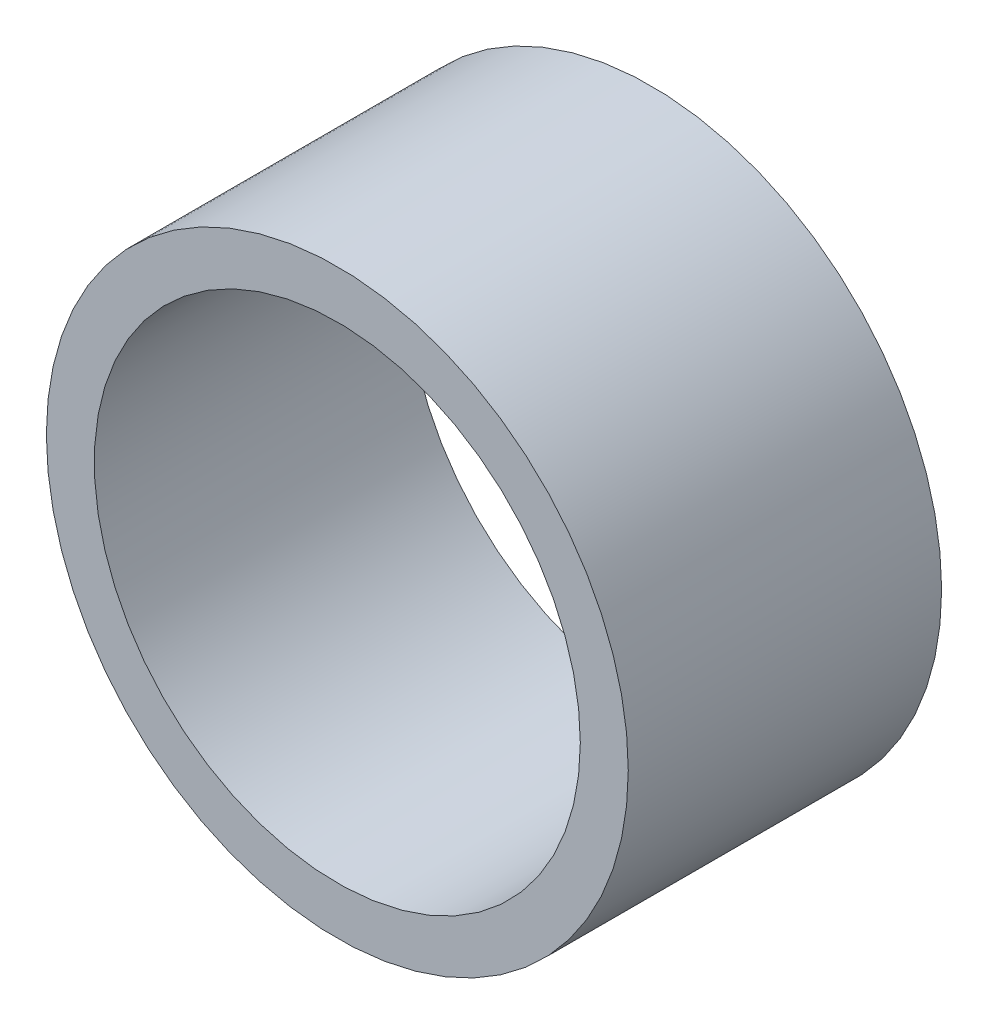
# Autodesk Inventor part: spacer for top of drivetrain
Saved by Autodesk Inventor 2020 (Build 240168000, 168)
## iProperties
Created: 2020-02-27
Part Number: spacer for top of drivetrain
Material: Generic
Document SubType Name: Modeling
Designer: jackm
Density: 1 g/cm^3
Appearance: Default
Author: jackm
Autodesk Inventor part; units mm, degrees
ref_plane "YZ Plane" through (0, 0, 0) normal (1, 0, 0) x (0, 1, 0)
ref_plane "XZ Plane" through (0, 0, 0) normal (0, 1, 0) x (-1, 0, 0)
ref_plane "XY Plane" through (0, 0, 0) normal (0, 0, 1) x (1, 0, 0)
ref_plane "Work Plane1" through (255.2636, 100.7805, 0) normal (0, 0, 1) x (1, 0, 0)
sketch "Sketch1" plane through (255.2636, 100.7805, 0) normal (0, 0, 1) x (1, 0, 0)
  arc A0 (-261.7645, -84.273) -> (-262.7946, -85.3989) centre (-263.6436, -83.5881) ccw construction
  circle A1 centre (-263.6436, -83.5881) radius 1.9304
  circle A2 centre (-263.6436, -83.5881) radius 2.3114
  point P0 (-255.2636, -100.7805)
  dimension "d0" = 3.8608
  dimension "d1" = 4.6228
  constraints: 2 centre point, 2 coincident
  measures "d0" diameter of A1
  measures "d1" diameter of A2
extrude "Extrusion1" add sketch "Sketch1" along normal blind 2.4892
body "Solid1"
